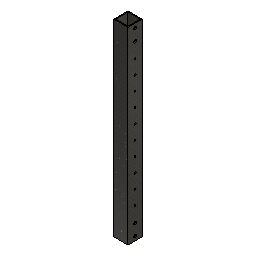
Vorbon Assembly (Autodesk Fusion 360 archive; units mm, degrees)
design "Carbon Tube"
Autodesk Fusion 360 part; units mm, degrees
sketch "Sketch1" plane through (0, 0, 0) normal (0, 0, 1) x (1, 0, 0)
  line L0 (7.5, 7.5) -> (-7.5, 7.5)
  line L1 (-7.5, 7.5) -> (-7.5, -7.5)
  line L2 (-7.5, -7.5) -> (7.5, -7.5)
  line L3 (7.5, -7.5) -> (7.5, 7.5)
  line L4 (7.5, 7.5) -> (-7.5, -7.5) construction
  line L5 (-7.5, 7.5) -> (7.5, -7.5) construction
  line L6 (6.5, 6.5) -> (-6.5, 6.5)
  line L7 (-6.5, 6.5) -> (-6.5, -6.5)
  line L8 (-6.5, -6.5) -> (6.5, -6.5)
  line L9 (6.5, -6.5) -> (6.5, 6.5)
  line L10 (6.5, 6.5) -> (-6.5, -6.5) construction
  line L11 (-6.5, 6.5) -> (6.5, -6.5) construction
  dimension "d1" = 15
  dimension "d2" = 15
  dimension "d3" = 13
  dimension "d4" = 13
  constraint horizontal L0
  constraint perpendicular L0 L1
  constraint parallel L0 L2
  constraint parallel L1 L3
  constraint coincident L4 origin
  constraint coincident L5 origin
  constraint horizontal L6
  constraint perpendicular L6 L7
  constraint parallel L6 L8
  constraint parallel L7 L9
  constraint coincident L10 origin
  constraint coincident L11 origin
  measures "d1" distance of L1.end L2.end
  measures "d2" distance of L0.end L1.end
  measures "d3" distance of L7.end L8.end
  measures "d4" distance of L6.end L7.end
extrude "Extrude1" add sketch "Sketch1" along normal blind 200
sketch "Sketch2" plane through (7.5, 0, 0) normal (1, 0, 0) x (0, 1, 0)
  line L0 (-7.5, 0) -> (7.5, 0)
  line L1 (7.5, 0) -> (7.5, 200)
  line L2 (7.5, 200) -> (-7.5, 200)
  line L3 (-7.5, 200) -> (-7.5, 0)
  circle A0 centre (0, 4.5) radius 1.5
  circle A1 centre (0, 16.5) radius 1.5
  circle A2 centre (0, 32.5) radius 1
  circle A3 centre (0, 47.5) radius 1
  circle A4 centre (0, 62.5) radius 1
  circle A5 centre (0, 77.5) radius 1
  circle A6 centre (0, 92.5) radius 1
  circle A7 centre (0, 107.5) radius 1
  circle A8 centre (0, 122.5) radius 1
  circle A9 centre (0, 137.5) radius 1
  circle A10 centre (0, 152.5) radius 1
  circle A11 centre (0, 167.5) radius 1
  circle A12 centre (0, 195.5) radius 1.5
  circle A13 centre (0, 183.5) radius 1.5
  dimension "d7" = 3
  dimension "d8" = 4.5
  dimension "d9" = 16.5
  dimension "d11" = 32.5
  dimension "d12" = 2
  dimension "d15" = 0
  dimension "d16" = 15
  dimension "d17" = 4.5
  dimension "d18" = 16.5
  dimension "d19" = 3
  dimension "d20" = 3
  constraint vertical origin A0.centre
  constraint vertical origin A1.centre
  constraint equal A0 A1
  constraint vertical origin A2.centre
  constraint vertical origin A12.centre
  constraint vertical origin A13.centre
  measures "d7" diameter of A0
  measures "d8" distance of L0 A0.centre
  measures "d9" distance of L0 A1.centre
  measures "d11" distance of L0 A2.centre
  measures "d12" diameter of A2
  measures "d17" distance of L2 A12.centre
  measures "d18" distance of L2 A13.centre
  measures "d19" diameter of A13
  measures "d20" diameter of A12
extrude "Extrude2" cut sketch "Sketch2" against normal blind 5 contours A0 | A1 | A2 | A3 | A4 | A5 | A6 | A7 | A8 | A9 | A10 | A11 | A12 | A13
extrude "Extrude3" cut sketch "Sketch2" against normal blind 25 contours A1 | A13
